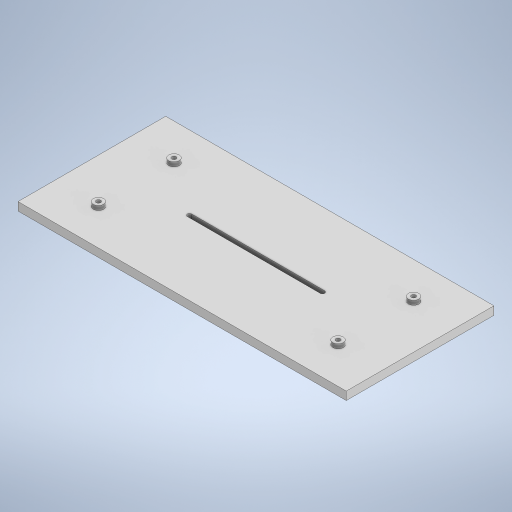
# Autodesk Inventor part: battery holder v2 mount
Saved by Autodesk Inventor 2023 (Build 270158000, 158)
## iProperties
Created: 2023-01-18
Part Number: battery holder v2 mount
Material: Generic
Document SubType Name: Modeling
Designer: agent
Density: 1 g/cm^3
Appearance: Default
Author: agent
Autodesk Inventor part; units mm, degrees
ref_plane "YZ Plane" through (0, 0, 0) normal (1, 0, 0) x (0, 1, 0)
ref_plane "XZ Plane" through (0, 0, 0) normal (0, 1, 0) x (-1, 0, 0)
ref_plane "XY Plane" through (0, 0, 0) normal (0, 0, 1) x (1, 0, 0)
sketch "Sketch1" plane through (0, 0, 0) normal (0, 1, 0) x (-1, 0, 0)
  circle A0 centre (113.7717, -57.4772) radius 1.35
  circle A1 centre (113.7717, -103.4772) radius 1.35
  circle A2 centre (-32.2283, -57.4772) radius 1.35
  circle A3 centre (-32.2283, -103.4772) radius 1.35
  line L0 (140.7717, -35.4772) -> (-59.2283, -35.4772)
  line L1 (-59.2283, -35.4772) -> (-59.2283, -125.4772)
  line L2 (-59.2283, -125.4772) -> (140.7717, -125.4772)
  line L3 (140.7717, -125.4772) -> (140.7717, -35.4772)
  point P0 (0, 0)
  point P1 (140.7717, -80.4772)
  dimension "d2" = 2.7
  dimension "d3" = 2.7
  dimension "d4" = 2.7
  dimension "d5" = 2.7
  dimension "d6" = 200
  dimension "d7" = 90
  constraints: 8 end point, 4 centre point, 2 parallel, 1 horizontal, 1 midpoint, 1 perpendicular
  measures "d2" diameter of A0
  measures "d3" diameter of A1
  measures "d4" diameter of A2
  measures "d5" diameter of A3
  measures "d6" distance of L2.end L1.end
  measures "d7" distance of L1.end L0.end
extrude "Extrusion1" add sketch "Sketch1" along normal blind 5
sketch "Sketch2" plane through (0, 5, 0) normal (0, 1, 0) x (1, 0, 0)
  circle A0 centre (-72.5219, 80.4772) radius 1.35
  circle A1 centre (-9.0219, 80.4772) radius 1.35
  circle A2 centre (-40.7719, 80.4772) radius 1.35
  line L0 (-140.7717, 125.4772) -> (-140.7717, 35.4772) projected
  point P0 (0, 0)
  point P1 (-140.7717, 80.4772)
  dimension "d12" = 2.7
  dimension "d13" = 2.7
  dimension "d14" = 63.5
  dimension "d15" = 2.7
  dimension "d16" = 31.75
  dimension "d22" = 68.2498
  constraints: 3 centre point, 1 midpoint
  measures "d12" diameter of A0
  measures "d13" diameter of A1
  measures "d14" distance of A1.centre A0.centre
  measures "d15" diameter of A2
  measures "d16" distance of A0.centre A2.centre
  measures "d22" distance of point (-140.772, 80.477) A0.centre
extrude "Extrusion2" cut sketch "Sketch2" against normal blind 11.35
sketch "Sketch3" plane through (0, 5, 0) normal (0, 1, 0) x (1, 0, 0)
  circle A0 centre (-113.7717, 57.4772) radius 1.35 projected
  circle A1 centre (-113.7717, 57.4772) radius 3.175
  circle A2 centre (-113.7717, 57.4772) radius 1.35
  circle A3 centre (-113.7717, 103.4772) radius 1.35 projected
  circle A4 centre (-113.7717, 103.4772) radius 1.35
  circle A5 centre (-113.7717, 103.4772) radius 3.175
  circle A6 centre (32.2283, 103.4772) radius 1.35 projected
  circle A7 centre (32.2283, 103.4772) radius 1.35
  circle A8 centre (32.2283, 103.4772) radius 3.175
  circle A9 centre (32.2283, 57.4772) radius 1.35 projected
  circle A10 centre (32.2283, 57.4772) radius 1.35
  circle A11 centre (32.2283, 57.4772) radius 3.175
  point P0 (0, 0)
  dimension "d25" = 6.35
  dimension "d26" = 6.35
  dimension "d27" = 6.35
  dimension "d28" = 6.35
  constraints: 8 centre point, 8 coincident, 1 concentric
  measures "d25" diameter of A1
  measures "d26" diameter of A5
  measures "d27" diameter of A8
  measures "d28" diameter of A11
extrude "Extrusion3" add sketch "Sketch3" along normal blind 2.54 contours A0 | A1 | A3 | A5 | A6 | A8 | A9 | A11
sketch "Sketch4" plane through (-113.7717, 7.54, -57.4772) normal (0, 1, 0) x (1, 0, 0)
  circle A0 centre (0, 0) radius 1.35 projected
  circle A1 centre (0, 0) radius 1.35
  circle A2 centre (0, 46) radius 1.35 projected
  circle A3 centre (0, 46) radius 1.35
  circle A4 centre (146, 46) radius 1.35 projected
  circle A5 centre (146, 46) radius 1.35
  circle A6 centre (146, 0) radius 3.175 projected
  circle A7 centre (146, 0) radius 1.35
  point P0 (113.7717, -57.4772)
  dimension "d31" = 2.7
  dimension "d32" = 2.7
  dimension "d33" = 2.7
  dimension "d34" = 2.7
  constraints: 4 centre point, 4 coincident
  measures "d31" diameter of A1
  measures "d32" diameter of A3
  measures "d33" diameter of A5
  measures "d34" diameter of A7
extrude "Extrusion4" cut sketch "Sketch4" against normal blind 21.59 contours A0 | A2 | A4 | A7
sketch "Sketch5" plane through (0, 5, 0) normal (0, 1, 0) x (1, 0, 0)
  circle A0 centre (-72.5219, 80.4772) radius 1.35 projected
  circle A1 centre (-9.0219, 80.4772) radius 1.35 projected
  line L0 (-72.5219, 79.1272) -> (-9.0219, 79.1272)
  line L1 (-9.0219, 79.1272) -> (-9.0219, 81.8272)
  line L2 (-9.0219, 81.8272) -> (-72.5219, 81.8272)
  line L3 (-72.5219, 81.8272) -> (-72.5219, 79.1272)
  line L4 (-72.5219, 81.8272) -> (-81.2922, 81.8272)
  line L5 (-81.2922, 81.8272) -> (-81.2922, 79.1272)
  line L6 (-81.2922, 79.1272) -> (-72.5219, 79.1272)
  line L7 (-72.5219, 79.1272) -> (-72.5219, 81.8272)
  line L8 (-9.0219, 81.8272) -> (-0.2589, 81.8272)
  line L9 (-0.2589, 81.8272) -> (-0.2589, 79.1272)
  line L10 (-0.2589, 79.1272) -> (-9.0219, 79.1272)
  line L11 (-9.0219, 79.1272) -> (-9.0219, 81.8272)
  circle A2 centre (-81.2922, 80.4772) radius 1.35
  circle A3 centre (-0.2589, 80.4772) radius 1.35
  point P0 (0, 0)
  dimension "d37" = 8.763
  dimension "d38" = 8.7702
  constraints: 24 end point, 6 parallel, 3 horizontal, 3 perpendicular, 2 midpoint, 2 point on line, 1 vertical alignment, 9 other
  measures "d37" distance of L9.end L10.end
  measures "d38" distance of L5.end L0.start
extrude "Extrusion5" cut sketch "Sketch5" against normal up to surface (5 mm away) contours A0 L3 | A0 L2 A1 L0 | L3 A0 | A0 L6 A2 L4 | L8 A3 L10 A1 | A2 L5 | L5 A2 | A3 L9 | L9 A3
body "Solid1"
